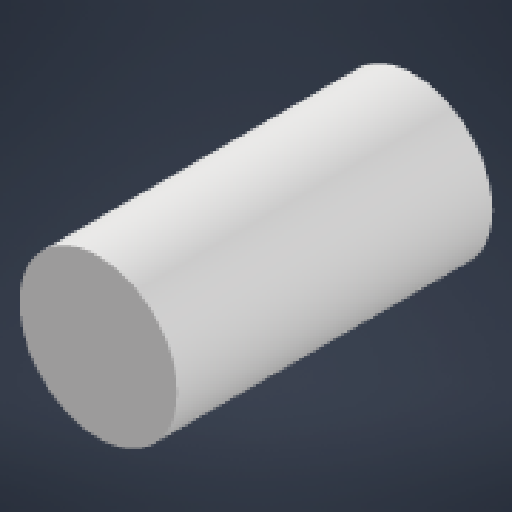
# Autodesk Inventor part: claw_static_mount_rod
Saved by Autodesk Inventor 2026 (Build 300175000, 175)
## iProperties
Created: 2025-03-27
Part Number: claw_static_mount_rod
Material: Generic
Document SubType Name: Modeling
Designer: paris
Density: 1 g/cm^3
Appearance: Default
Author: paris
Autodesk Inventor part; units mm, degrees
ref_plane "YZ Plane" through (0, 0, 0) normal (1, 0, 0) x (0, 1, 0)
ref_plane "XZ Plane" through (0, 0, 0) normal (0, 1, 0) x (-1, 0, 0)
ref_plane "XY Plane" through (0, 0, 0) normal (0, 0, 1) x (1, 0, 0)
sketch "Sketch1" plane through (0, 0, 0) normal (0, 0, 1) x (1, 0, 0)
  circle A0 centre (-20, 10) radius 2.5 projected
  circle A1 centre (0, -5) radius 2.5 projected
  circle A2 centre (-20, -10) radius 2.5 projected
  circle A3 centre (0, 5) radius 2.5 projected
  line L0 (28.75, 10) -> (28.75, -10) projected
  line L1 (28.75, 10) -> (-8.2322, 10) projected
  line L2 (-10, 11.25) -> (-8.2322, 10) projected
  line L3 (-10, 11.25) -> (-10, 16.25) projected
  line L4 (-28.75, 16.25) -> (-10, 16.25) projected
  line L5 (-28.75, -16.25) -> (-28.75, 16.25) projected
  line L6 (-10, -16.25) -> (-28.75, -16.25) projected
  line L7 (-10, -16.25) -> (-10, -11.25) projected
  line L8 (-8.2322, -10) -> (-10, -11.25) projected
  line L9 (-8.2322, -10) -> (28.75, -10) projected
  point P0 (0, 0)
extrude "Extrusion1" add sketch "Sketch1" against normal blind 10 contours A2
body "Solid1"
